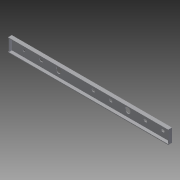
# Autodesk Inventor part: MICHAUD CHAILLY B3 - 21 - 30 - 2
Saved by Autodesk Inventor 2011 SP1 (Build 150282100, 282)
## iProperties
Created: 2012-12-20
Part Number: MICHAUD CHAILLY B3 - 21 - 30 - 2
Catalog Web Link: www.cadenas.de
Description: Modèle B3-21-2-GLISSIERE DOUBLE COURSE 75%
Vendor: EMILEMAURIN
Document SubType Name: Modeling
Designer: PARTuser1
Manufacturer: EMILEMAURIN
Density: 1 g/cm^3
Category: PARTsolutions
Company: EMILEMAURIN
Title: MICHAUD CHAILLY B3 - 21 - 30 - 2
Author: Cadenas PARTsolutions
Comments: GLISSIERE DOUBLE COURSE 75%
PSOL_IDENT_0: {\\10.0.0.242\data_v9\23d-libs\michaud_chailly_transmission\guidage\autres_composants\glissieres_a_b
PSOL_IDENT_1: illes\b3_21\b3_21_2.prj},214 {VTYP=3D},{NB=MICHAUD CHAILLY B3 - 21 - 30 - 2},{LINA=MICHAUD CHAILLY B
PSOL_IDENT_2: 3 - 21 - 30 - 2},{NN=Modèle B3-21-2},{DATE=11.03.2011 14:16:37},{GEOMDATE=10.04.2007 10:35:00},{VERS
PSOL_IDENT_3: ION=},{LINEID=20},{LINESUBID=-1},{WBVAR=}  {NB=michaud_chailly_B3 - 21 - 30_2},{LINA=MICHAUD CHAILLY
PSOL_IDENT_4: B3 - 21 - 30 - 2},{KT=DUMMY},{REF=B3 - 21 - 30},{L=295},{L1=150.300},{L2=182.300},{L3=246.300},{L4=
PSOL_IDENT_5: 278.300},{L5=87.500},{L6=215.000}
CNS_NT: GLISSIERE DOUBLE COURSE 75%
CNS_NB: michaud_chailly_B3 - 21 - 30_2
CNS_NBSYN: michaud_chailly_$REF._2
CNS_LINA: MICHAUD CHAILLY B3 - 21 - 30 - 2
CNS_REF: B3 - 21 - 30
CNS_L: 295
CNS_L1: 150.300
CNS_L2: 182.300
CNS_L3: 246.300
CNS_L4: 278.300
CNS_L5: 87.500
CNS_L6: 215.000
SUPPLIER: EMILEMAURIN
ARTICLENO: MICHAUD CHAILLY B3 - 21 - 30 - 2
BOMINFO: MICHAUD CHAILLY B3 - 21 - 30 - 2
CREATOR: CADENAS GmbH
Autodesk Inventor part; units mm, degrees
sketch "Esquisse_1" plane through (0, 0, 0) normal (1, 0, 0) x (0, 1, 0)
  line L0 (2.6, 12.15) -> (2.6, 10.9)
  line L1 (2.6, 10.9) -> (8.25, 10.9)
  line L2 (8.25, 10.9) -> (8.25, -10.9)
  line L3 (8.25, -10.9) -> (2.6, -10.9)
  line L4 (2.6, -10.9) -> (2.6, -12.15)
  line L5 (2.6, -12.15) -> (9.5, -12.15)
  line L6 (9.5, -12.15) -> (9.5, 12.15)
  line L7 (9.5, 12.15) -> (2.6, 12.15)
  constraints: 16 end point
extrude "Extrusion1" add sketch "Esquisse_1" along normal blind 295
sketch "Esquisse_2" plane through (0, 0, 0) normal (1, 0, 0) x (0, 1, 0)
  line L0 (9.5, 10.9) -> (3.5, 10.9)
  line L1 (3.5, 10.9) -> (3.5, -10.9)
  line L2 (3.5, -10.9) -> (9.5, -10.9)
  line L3 (9.5, -10.9) -> (9.5, 10.9)
  constraints: 8 end point
extrude "Extrusion2" add sketch "Esquisse_2" along normal blind 1.5
sketch "Esquisse_3" plane through (295, 0, 0) normal (1, 0, 0) x (0, 0, -1)
  line L0 (-10.9, 9.5) -> (-10.9, 3.5)
  line L1 (-10.9, 3.5) -> (10.9, 3.5)
  line L2 (10.9, 3.5) -> (10.9, 9.5)
  line L3 (10.9, 9.5) -> (-10.9, 9.5)
  constraints: 8 end point
extrude "Extrusion3" add sketch "Esquisse_3" against normal blind 1.5
sketch "Esquisse_4" plane through (0, 0, 0) normal (0, 1, 0) x (-1, 0, 0)
  circle A0 centre (-23.4, 0) radius 2.15
  constraints: 1 centre point
extrude "Extrusion4" cut sketch "Esquisse_4" along normal blind 9.5
sketch "Esquisse_5" plane through (0, 0, 0) normal (0, 1, 0) x (-1, 0, 0)
  arc A0 (-54.3, -2.15) -> (-54.3, 2.15) centre (-54.3, 0) ccw
  line L0 (-54.3, 2.15) -> (-56.5, 2.15)
  arc A1 (-56.5, 2.15) -> (-56.5, -2.15) centre (-56.5, 0) ccw
  line L1 (-56.5, -2.15) -> (-54.3, -2.15)
  constraints: 4 end point, 4 point on circle, 2 centre point
extrude "Extrusion5" cut sketch "Esquisse_5" along normal blind 9.5
sketch "Esquisse_6" plane through (0, 0, 0) normal (0, 1, 0) x (-1, 0, 0)
  arc A0 (-150.3, -2.15) -> (-150.3, 2.15) centre (-150.3, 0) ccw
  line L0 (-150.3, 2.15) -> (-152.5, 2.15)
  arc A1 (-152.5, 2.15) -> (-152.5, -2.15) centre (-152.5, 0) ccw
  line L1 (-152.5, -2.15) -> (-150.3, -2.15)
  constraints: 4 end point, 4 point on circle, 2 centre point
extrude "Extrusion6" cut sketch "Esquisse_6" along normal blind 9.5
sketch "Esquisse_7" plane through (0, 0, 0) normal (0, 1, 0) x (-1, 0, 0)
  arc A0 (-182.3, -2.15) -> (-182.3, 2.15) centre (-182.3, 0) ccw
  line L0 (-182.3, 2.15) -> (-184.5, 2.15)
  arc A1 (-184.5, 2.15) -> (-184.5, -2.15) centre (-184.5, 0) ccw
  line L1 (-184.5, -2.15) -> (-182.3, -2.15)
  constraints: 4 end point, 4 point on circle, 2 centre point
extrude "Extrusion7" cut sketch "Esquisse_7" along normal blind 9.5
sketch "Esquisse_8" plane through (0, 0, 0) normal (0, 1, 0) x (-1, 0, 0)
  arc A0 (-246.3, -2.15) -> (-246.3, 2.15) centre (-246.3, 0) ccw
  line L0 (-246.3, 2.15) -> (-248.5, 2.15)
  arc A1 (-248.5, 2.15) -> (-248.5, -2.15) centre (-248.5, 0) ccw
  line L1 (-248.5, -2.15) -> (-246.3, -2.15)
  constraints: 4 end point, 4 point on circle, 2 centre point
extrude "Extrusion8" cut sketch "Esquisse_8" along normal blind 9.5
sketch "Esquisse_9" plane through (0, 0, 0) normal (0, 1, 0) x (-1, 0, 0)
  arc A0 (-278.3, -2.15) -> (-278.3, 2.15) centre (-278.3, 0) ccw
  line L0 (-278.3, 2.15) -> (-280.5, 2.15)
  arc A1 (-280.5, 2.15) -> (-280.5, -2.15) centre (-280.5, 0) ccw
  line L1 (-280.5, -2.15) -> (-278.3, -2.15)
  constraints: 4 end point, 4 point on circle, 2 centre point
extrude "Extrusion9" cut sketch "Esquisse_9" along normal blind 9.5
sketch "Esquisse_10" plane through (0, 0, 0) normal (0, 1, 0) x (-1, 0, 0)
  circle A0 centre (-87.5, 0) radius 5
  constraints: 1 centre point
extrude "Extrusion10" cut sketch "Esquisse_10" along normal blind 9.5
sketch "Esquisse_11" plane through (0, 0, 0) normal (0, 1, 0) x (-1, 0, 0)
  circle A0 centre (-215, 0) radius 5
  constraints: 1 centre point
extrude "Extrusion11" cut sketch "Esquisse_11" along normal blind 9.5
ref_plane "IP0_XY" through (0, 0, 0) normal (1, 0, 0) x (0, 0, -1)
ref_plane "IP0_YZ" through (0, 0, 0) normal (0, 0, -1) x (0, 1, 0)
ref_plane "IP0_ZX" through (0, 0, 0) normal (0, 1, 0) x (1, 0, 0)
body "Solid1"
